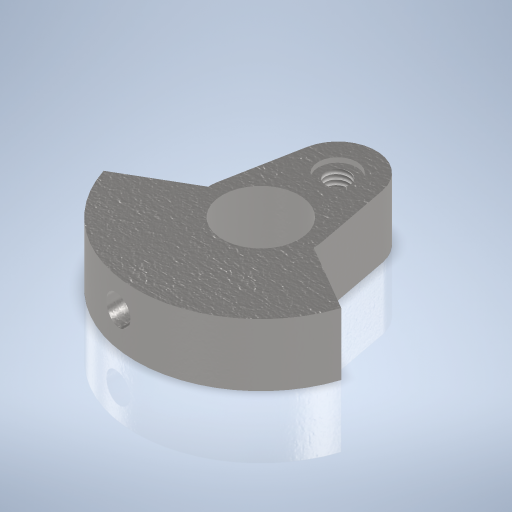
# Autodesk Inventor part: Kurbel
Saved by Autodesk Inventor 2024 (Build 280153000, 153)
## iProperties
Created: 2024-01-15
Part Number: Kurbel
Material: Stahl, galvanisiert
Document SubType Name: Modeling
Designer: ffogue
Density: 7.85 g/cm^3
Appearance: Galvanisiert
Author: ffogue
Autodesk Inventor part; units mm, degrees
ref_plane "YZ Plane" through (0, 0, 0) normal (1, 0, 0) x (0, 1, 0)
ref_plane "XY Plane" through (0, 0, 0) normal (0, 0, 1) x (1, 0, 0)
sketch "Skizze1" plane through (0, 0, 0) normal (0, 0, 1) x (1, 0, 0)
  line L0 (-2.6307, 4) -> (27.3693, 4) construction
  arc A0 (0, 0) -> (24.7386, 0) centre (12.3693, 4) ccw
  circle A1 centre (12.3693, 4) radius 5.5
  line L1 (17.8693, 4) -> (24.7386, 0)
  line L2 (6.8693, 4) -> (0, 0)
  line L3 (6.9669, 5.0312) -> (8.4403, 12.75)
  line L4 (17.7718, 5.0312) -> (16.2984, 12.75)
  arc A2 (16.2984, 12.75) -> (8.4403, 12.75) centre (12.3693, 12) ccw
  dimension "d2" = 26
  dimension "d3" = 11
  dimension "d4" = 4
  dimension "d5" = 4
  dimension "d6" = 8
  constraints: 10 end point, 8 point on circle, 4 tangent, 3 centre point, 2 coincident, 2 point on line, 1 equal length, 1 horizontal, 1 midpoint, 1 vertical alignment
  measures "d2" diameter of A0
  measures "d3" diameter of A1
  measures "d4" distance from line of L1.end L0
  measures "d5" radius of A2
  measures "d6" distance of A2.centre A0.centre
extrude "Extrusion1" add sketch "Skizze1" along normal blind 6.5
sketch "Skizze2" plane through (0, 0, 6.5) normal (0, 0, 1) x (1, 0, 0)
  arc A0 (17.8693, 4) -> (17.7718, 5.0312) centre (12.3693, 4) ccw projected
  line L0 (17.7718, 5.0312) -> (16.2984, 12.75) projected
  arc A1 (16.2984, 12.75) -> (8.4403, 12.75) centre (12.3693, 12) ccw projected
  line L1 (8.4403, 12.75) -> (6.9669, 5.0312) projected
  arc A2 (6.9669, 5.0312) -> (6.8693, 4) centre (12.3693, 4) ccw projected
  line L2 (6.8693, 4) -> (0, 0) projected
  arc A3 (0, 0) -> (24.7386, 0) centre (12.3693, 4) ccw projected
  line L3 (24.7386, 0) -> (17.8693, 4) projected
  circle A4 centre (12.3693, 4) radius 4
  dimension "d9" = 8
  constraints: 1 centre point, 1 coincident
  measures "d9" diameter of A4
extrude "Extrusion2" cut sketch "Skizze2" against normal up to surface (6.5 mm away) contours A4
sketch "Skizze3" plane through (0, 0, 6.5) normal (0, 0, 1) x (1, 0, 0)
  circle A0 centre (12.3693, 4) radius 4 projected
  point P0 (0, 0)
  point P1 (12.3693, 12)
  dimension "d12" = 8
  constraints: 1 vertical alignment
  measures "d12" distance of A0.centre point (12.369, 12)
hole "Bohrung1" at (12.3693, 12, 6.5) direction (0, 0, -1) diameter 2.459 depth 6.5 counterbore diameter 4 counterbore depth 0.5 thread size "M3x0.5" class "6H" standard "ISO Metric profile"
ref_plane "Arbeitsebene1" through (0, 0, 0) normal (0, 1, 0) x (-1, 0, 0)
sketch "Skizze4" plane through (0, 0, 0) normal (0, 1, 0) x (-1, 0, 0)
  line L0 (0, 6.5) -> (-24.7386, 6.5) projected
  line L1 (0, 0) -> (-24.7386, 0) projected
  line L2 (-24.7386, 0) -> (-24.7386, 6.5) projected
  line L3 (0, 6.5) -> (-24.7386, 6.5) projected
  line L4 (0, 0) -> (0, 6.5) projected
  point P0 (-12.3693, 6.5)
  point P1 (-10.2818, 3.5)
  point P2 (-12.3693, 6.5)
  dimension "d25" = 3
  dimension "d26" = 14.4568
  constraints: 2 midpoint
  measures "d25" distance from line of L0 point (-10.282, 3.5)
  measures "d26" distance from line of L2 point (-10.282, 3.5)
hole "Bohrung2" at (10.2818, 0, 3.5) direction (0, -1, 0) diameter 3 end through all
